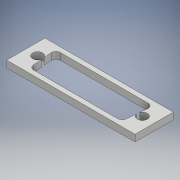
# Autodesk Inventor part: Eletronica - Com25pin
Saved by Autodesk Inventor 2017 (Build 210142000, 142)
## iProperties
Created: 2020-08-30
Part Number: Eletronica - Com25pin
Material: Generic
Document SubType Name: Modeling
Designer: ale
Density: 1 g/cm^3
Appearance: Default
Author: ale
Autodesk Inventor part; units mm, degrees
ref_plane "YZ Plane" through (0, 0, 0) normal (1, 0, 0) x (0, 1, 0)
ref_plane "XZ Plane" through (0, 0, 0) normal (0, 1, 0) x (-1, 0, 0)
ref_plane "XY Plane" through (0, 0, 0) normal (0, 0, 1) x (1, 0, 0)
sketch "Sketch1" plane through (0, 0, 0) normal (0, 0, 1) x (1, 0, 0)
  line L0 (19.5024, 6.36) -> (-19.5024, 6.36)
  arc A0 (-19.5024, 6.36) -> (-21.4937, 4.1742) centre (-19.5024, 4.36) ccw
  line L1 (-21.4937, 4.1742) -> (-20.6803, -4.5458)
  arc A1 (-20.6803, -4.5458) -> (-18.6889, -6.36) centre (-18.6889, -4.36) ccw
  line L2 (-18.6889, -6.36) -> (18.6889, -6.36)
  arc A2 (18.6889, -6.36) -> (20.6803, -4.5458) centre (18.6889, -4.36) ccw
  line L3 (20.6803, -4.5458) -> (21.4937, 4.1742)
  arc A3 (21.4937, 4.1742) -> (19.5024, 6.36) centre (19.5024, 4.36) ccw
  line L4 (-28.5, 8.5) -> (28.5, 8.5)
  line L5 (28.5, 8.5) -> (28.5, -8.5)
  line L6 (28.5, -8.5) -> (-28.5, -8.5)
  line L7 (-28.5, -8.5) -> (-28.5, 8.5)
  arc A4 (-21.1884, 0.9013) -> (-21.0573, -0.5045) centre (-23.25, 0) ccw
  arc A5 (21.0573, -0.5045) -> (21.1884, 0.9013) centre (23.25, 0) ccw
  point P0 (19.6, -5.36)
  point P1 (-19.6, -5.36)
  dimension "d2" = 39.2
  dimension "d9" = 57
  dimension "d10" = 17
  constraints: 16 end point, 12 point on circle, 6 centre point, 4 point on line, 3 parallel, 1 horizontal, 1 perpendicular
  measures "d2" distance of point (19.6, -5.36) point (-19.6, -5.36)
  measures "d9" distance of L5.end L6.end
  measures "d10" distance of L4.end L5.end
extrude "Extrusion1" add sketch "Sketch1" along normal blind 3
body "Solid1"
